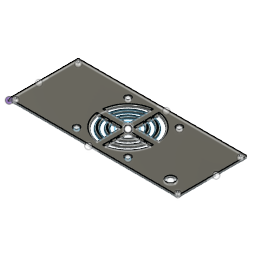
Resistor Box Back Panel (Autodesk Fusion 360 design; units mm, degrees)
Autodesk Fusion 360 part; units mm, degrees
sketch "Sketch1" plane through (0, 0, 0) normal (0, 0, 1) x (1, 0, 0)
  line L0 (0, 0) -> (234.75, 0)
  line L1 (234.75, 0) -> (234.75, 96.2)
  line L2 (234.75, 96.2) -> (0, 96.2)
  line L3 (0, 96.2) -> (0, 0)
  circle A0 centre (4.3, 91.9) radius 1.5625
  circle A1 centre (230.45, 91.9) radius 1.5625
  circle A2 centre (230.45, 4.3) radius 1.5625
  circle A3 centre (4.3, 4.3) radius 1.5625
  circle A4 centre (209.75, 15) radius 6.375
  circle A5 centre (81.625, 83.85) radius 2.6
  circle A6 centre (153.125, 83.85) radius 2.6
  circle A7 centre (81.6225, 12.35) radius 2.6
  circle A8 centre (153.1225, 12.35) radius 2.6
  line L4 (110.5, 96.2) -> (122.5, 96.2)
  line L5 (122.5, 0) -> (110.5, 0)
  line L6 (234.75, 53.5) -> (234.75, 41.5)
  line L7 (0, 41.5) -> (0, 53.5)
  arc A9 (111.375, 59.1164) -> (106.3586, 54.1) centre (117.375, 48.1) ccw
  arc A10 (105.725, 42.1) -> (111.375, 36.45) centre (117.375, 48.1) ccw
  arc A11 (111.375, 64.5492) -> (100.9258, 54.1) centre (117.375, 48.1) ccw
  arc A12 (100.2793, 42.1) -> (111.375, 31.0043) centre (117.375, 48.1) ccw
  arc A13 (111.375, 69.7734) -> (95.7016, 54.1) centre (117.375, 48.1) ccw
  arc A14 (95.0491, 42.1) -> (111.375, 25.7741) centre (117.375, 48.1) ccw
  arc A15 (111.375, 74.9121) -> (90.5629, 54.1) centre (117.375, 48.1) ccw
  arc A16 (89.9068, 42.1) -> (111.375, 20.6318) centre (117.375, 48.1) ccw
  arc A17 (111.375, 80.0068) -> (85.4682, 54.1) centre (117.375, 48.1) ccw
  arc A18 (84.8098, 42.1) -> (111.375, 15.5348) centre (117.375, 48.1) ccw
  arc A19 (111.375, 85.1169) -> (111.375, 11.0831) centre (117.375, 48.1) ccw
  arc A20 (123.375, 11.0831) -> (154.3919, 42.1) centre (117.375, 48.1) ccw
  arc A21 (154.3919, 54.1) -> (123.375, 85.1169) centre (117.375, 48.1) ccw
  arc A22 (123.375, 16.1586) -> (149.3164, 42.1) centre (117.375, 48.1) ccw
  arc A23 (148.7048, 54.1) -> (123.375, 79.4298) centre (117.375, 48.1) ccw
  arc A24 (123.375, 21.2625) -> (144.2125, 42.1) centre (117.375, 48.1) ccw
  arc A25 (143.5957, 54.1) -> (123.375, 74.3207) centre (117.375, 48.1) ccw
  arc A26 (123.375, 26.4148) -> (139.0602, 42.1) centre (117.375, 48.1) ccw
  arc A27 (138.4352, 54.1) -> (123.375, 69.1602) centre (117.375, 48.1) ccw
  arc A28 (123.375, 31.6607) -> (133.8143, 42.1) centre (117.375, 48.1) ccw
  arc A29 (133.1743, 54.1) -> (123.375, 63.8993) centre (117.375, 48.1) ccw
  arc A30 (123.375, 37.1341) -> (128.3409, 42.1) centre (117.375, 48.1) ccw
  arc A31 (127.6661, 54.1) -> (123.375, 58.3911) centre (117.375, 48.1) ccw
  line L8 (123.375, 85.1169) -> (123.375, 54.1)
  line L9 (123.375, 42.1) -> (123.375, 11.0831)
  line L10 (111.375, 11.0831) -> (111.375, 42.1)
  line L11 (111.375, 54.1) -> (111.375, 85.1169)
  line L12 (154.3919, 42.1) -> (123.375, 42.1)
  line L13 (111.375, 42.1) -> (80.3581, 42.1)
  line L14 (80.3581, 54.1) -> (111.375, 54.1)
  line L15 (123.375, 54.1) -> (154.3919, 54.1)
  dimension "d1" = 234.75
  dimension "d2" = 96.2
  dimension "d3" = 3.125
  dimension "d4" = 4.3
  dimension "d5" = 4.3
  dimension "d6" = 4.3
  dimension "d7" = 4.3
  dimension "d8" = 4.3
  dimension "d9" = 4.3
  dimension "d10" = 4.3
  dimension "d11" = 4.3
  dimension "d16" = 12.75
  dimension "d17" = 25
  dimension "d18" = 15
  dimension "d27" = 5.2
  dimension "d28" = 71.5
  dimension "d29" = 71.5
  dimension "d30" = 71.5
  dimension "d31" = 71.5
  dimension "d32" = 81.625
  dimension "d33" = 12.35
  dimension "d34" = 48.1
  dimension "d35" = 117.375
  dimension "d36" = 75
  dimension "d37" = 65
  dimension "d38" = 55
  dimension "d39" = 45
  dimension "d40" = 35
  dimension "d41" = 25
  dimension "d42" = 6
  dimension "d43" = 6
  dimension "d44" = 6
  dimension "d45" = 6
  dimension "d54" = 12.35
  constraint horizontal L0
  constraint vertical L1
  constraint horizontal L2
  constraint vertical L3
  constraint coincident L0.start L3.end
  constraint equal A2 A3
  constraint equal A1 A2
  constraint equal A0 A1
  constraint equal A7 A8
  constraint equal A6 A8
  constraint equal A5 A6
  constraint concentric A20 A22
  constraint concentric A22 A24
  constraint concentric A20 A26
  constraint concentric A22 A28
  constraint concentric A24 A30
  constraint horizontal L4
  constraint vertical L8
  constraint horizontal L5
  constraint vertical L10
  constraint coincident L0 L5.start
  constraint coincident L2 L4.start
  constraint horizontal L14
  constraint vertical L6
  constraint horizontal L12
  constraint vertical L7
  constraint coincident L1 L6.end
  constraint coincident L3 L7.end
  constraint coincident A19.start A20
  constraint coincident L14.start A20
  constraint coincident L13.end A20
  constraint coincident A21.start A20
  constraint coincident A10.end L10
  constraint coincident A30.start L8
  constraint coincident A12.end L10
  constraint coincident A28.start L8
  constraint coincident A14.end L10
  constraint coincident A26.start L8
  constraint coincident A16.end L10
  constraint coincident A24.start L8
  constraint coincident A18.end L10
  constraint coincident A22.start L8
  constraint coincident A31.end L8
  constraint coincident A9.start L10
  constraint concentric A9 A30
  constraint coincident A29.end L8
  constraint coincident A11.start L10
  constraint concentric A11 A28
  constraint coincident A27.end L8
  constraint coincident A13.start L10
  constraint concentric A13 A26
  constraint coincident A25.end L8
  constraint coincident A15.start L10
  constraint concentric A15 A24
  constraint coincident A23.end L8
  constraint coincident A17.start L10
  constraint concentric A17 A22
  constraint coincident A9.end L14
  constraint coincident A10.start L12
  constraint concentric A9 A10
  constraint coincident A11.end L14
  constraint coincident A12.start L12
  constraint concentric A11 A12
  constraint coincident A13.end L14
  constraint coincident A14.start L12
  constraint concentric A13 A14
  constraint coincident A15.end L14
  constraint coincident A16.start L12
  constraint concentric A15 A16
  constraint coincident A17.end L14
  constraint coincident A18.start L12
  constraint concentric A17 A18
  constraint concentric A19 A20
  constraint concentric A20 A21
  constraint coincident A22.end L12
  constraint coincident A23.start L14
  constraint concentric A22 A23
  constraint coincident A24.end L12
  constraint coincident A25.start L14
  constraint concentric A24 A25
  constraint coincident A26.end L12
  constraint coincident A27.start L14
  constraint concentric A26 A27
  constraint coincident A28.end L12
  constraint coincident A29.start L14
  constraint concentric A28 A29
  constraint coincident A30.end L12
  constraint coincident A31.start L14
  constraint concentric A30 A31
  constraint coincident L8.end L14
  constraint collinear L8 L9
  constraint coincident L10.end L12
  constraint collinear L10 L11
  constraint collinear L12 L13
  constraint collinear L14 L15
  measures "d1" distance of L0.start L0.end
  measures "d2" distance of L0.start L2.end
  measures "d3" diameter of A0
  measures "d4" distance of L2 A0.centre
  measures "d5" distance of L3 A0.centre
  measures "d6" distance of L0 A3.centre
  measures "d7" distance of L3 A3.centre
  measures "d8" distance of L1 A2.centre
  measures "d9" distance of L0 A2.centre
  measures "d10" distance of L1 A1.centre
  measures "d11" distance of L2 A1.centre
  measures "d16" diameter of A4
  measures "d17" distance of L1 A4.centre
  measures "d18" distance of L0 A4.centre
  measures "d27" diameter of A5
  measures "d28" distance of A5.centre A6.centre
  measures "d29" distance of A7.centre A8.centre
  measures "d30" distance of A5.centre A7.centre
  measures "d31" distance of A6.centre A8.centre
  measures "d32" distance of L3 A5.centre
  measures "d33" distance of L2 A6.centre
  measures "d34" distance of L2 A9.centre
  measures "d35" distance of L3 A9.centre
  measures "d36" diameter of A20
  measures "d37" diameter of A22
  measures "d38" diameter of A24
  measures "d39" diameter of A26
  measures "d40" diameter of A28
  measures "d41" diameter of A30
  measures "d42" distance of A9.centre L10
  measures "d43" distance of A9.centre L8
  measures "d44" distance of A9.centre L14
  measures "d45" distance of A9.centre L12
  measures "d54" distance of L2 A5.centre
extrude "Extrude2" add sketch "Sketch1" along normal blind 2.5 contours L0 L1 L2 L3 L4 L5 L6 L7 | A11 A13 L11 L14 | A15 A17 L11 L14 | A12 A14 L10 L13 | A16 A18 L10 L13 | A22 A24 L9 L12 | A26 A28 L9 L12 | A23 A25 L8 L15 | A27 A29 L8 L15
chamfer "Chamfer2" distance 0.5 angle 45 4 edges at (234.75, 0, 1.25) (234.75, 96.2, 1.25) (0, 0, 1.25) (0, 96.2, 1.25)
fillet "Fillet1" radius 2 44 edges at (136.8204, 28.6546, 2.5) (140.356, 25.119, 2.5) (143.8915, 21.5835, 2.5) (151.8541, 42.1, 2.5) (151.5484, 54.1, 2.5) (143.8915, 74.6165, 2.5) (139.9311, 70.6561, 2.5) (136.395, 67.12, 2.5) (141.0154, 54.1, 2.5) (132.8594, 63.5844, 2.5) (141.6364, 42.1, 2.5) (133.2849, 32.1901, 2.5) (123.375, 23.8386, 2.5) (123.375, 13.6209, 2.5) (111.375, 13.3089, 2.5) (90.8585, 21.5835, 2.5) (93.9603, 24.6853, 2.5) (97.4941, 28.2191, 2.5) (101.028, 31.753, 2.5) (104.5636, 35.2886, 2.5) (111.375, 36.5522, 2.5) (105.8272, 42.1, 2.5) (123.375, 36.8804, 2.5) (129.7494, 35.7256, 2.5) (128.5946, 42.1, 2.5) (128.2747, 54.1, 2.5) (123.375, 58.9997, 2.5) (129.3253, 60.0503, 2.5) (123.375, 71.7404, 2.5) (123.375, 82.2734, 2.5) (111.375, 82.5619, 2.5) (111.375, 72.3427, 2.5) (104.994, 60.481, 2.5) (111.375, 59.3246, 2.5) (106.1504, 54.1, 2.5) (101.4732, 64.0018, 2.5) (93.1323, 54.1, 2.5) (97.9471, 67.5279, 2.5) (94.418, 71.057, 2.5) (90.8585, 74.6165, 2.5) (82.9131, 54.1, 2.5) (82.5839, 42.1, 2.5) (92.4779, 42.1, 2.5) (111.375, 23.2029, 2.5)
chamfer "Chamfer3" distance 1.5 angle 45 4 edges at (79.2009, 84.7902, 2.5) (150.7009, 84.7902, 2.5) (150.6984, 13.2902, 2.5) (79.1984, 13.2902, 2.5)
equation "d32 = ( ( 234.75 / 2 ) * 1 mm ) - ( 71.5 / 2 ) * 1 mm"
equation "d33 = ( ( 96.2 / 2 ) * 1 mm ) - ( 71.5 / 2 ) * 1 mm"
equation "d34 = ( 96.2 / 2 ) * 1 mm"
equation "d35 = ( 234.75 / 2 ) * 1 mm"
named bodies: "ResistorBX_BP"
